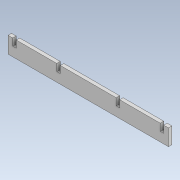
# Autodesk Inventor part: chassis_1_7
Saved by Autodesk Inventor 2022 (Build 260153000, 153)
## iProperties
Created: 2023-04-28
Part Number: chassis_1_7
Material: 一般
Document SubType Name: Modeling
Designer: Johnny Jou
Density: 1 g/cm^3
Appearance: 預設
Author: Johnny Jou
Autodesk Inventor part; units mm, degrees
ref_plane "YZ Plane" through (0, 0, 0) normal (1, 0, 0) x (0, 1, 0)
ref_plane "XZ Plane" through (0, 0, 0) normal (0, 1, 0) x (-1, 0, 0)
ref_plane "XY Plane" through (0, 0, 0) normal (0, 0, 1) x (1, 0, 0)
sketch "草圖1" plane through (0, 0, 0) normal (0, 0, 1) x (1, 0, 0)
  line L0 (0, 0) -> (124, 0)
  line L1 (124, 0) -> (124, -14) construction
  line L2 (124, -14) -> (0, -14)
  line L3 (0, -14) -> (0, 0) construction
  line L4 (35, 0) -> (37.95, 0)
  line L5 (37.95, 0) -> (37.95, -6)
  line L6 (37.95, -6) -> (35, -6)
  line L7 (35, -6) -> (35, 0)
  line L8 (89, 0) -> (86.05, 0)
  line L9 (86.05, 0) -> (86.05, -6)
  line L10 (86.05, -6) -> (89, -6)
  line L11 (89, -6) -> (89, 0)
  line L12 (131, -14) -> (126.95, -14)
  line L13 (124, 0) -> (131, 0)
  line L14 (131, 0) -> (131, -14)
  line L15 (126.95, -14) -> (126.95, -6)
  line L16 (126.95, -6) -> (124, -6)
  line L17 (0, 0) -> (-7, 0)
  line L18 (-7, 0) -> (-7, -14)
  line L19 (-7, -14) -> (-2.95, -14)
  line L20 (0, -14) -> (0, 0) construction
  line L21 (-2.95, -14) -> (-2.95, -6)
  line L22 (-2.95, -6) -> (0, -6)
  line L23 (0, -6) -> (0, -14)
  line L24 (124, -6) -> (124, -14)
  line L25 (124, -14) -> (126.95, -14)
  line L26 (124, -6) -> (126.95, -6)
  line L27 (126.95, -6) -> (126.95, 0)
  line L28 (126.95, 0) -> (124, 0)
  line L29 (124, 0) -> (124, -6)
  line L30 (-2.95, -14) -> (0, -14)
  line L31 (-2.95, -6) -> (0, -6)
  line L32 (0, -6) -> (0, 0)
  line L33 (0, 0) -> (-2.95, 0)
  line L34 (-2.95, 0) -> (-2.95, -6)
  point P0 (0, -15.5)
  point P1 (0, -6)
  point P2 (0, -14)
  dimension "d0" = 124
  dimension "d1" = 35
  dimension "d3" = 2.95
  dimension "d4" = 2.95
  dimension "d10" = 8
  dimension "d16" = 6
  dimension "d17" = 35
  dimension "d18" = 2.95
  dimension "d21" = 7
  dimension "d22" = 2.95
  dimension "d24" = 7
  dimension "d29" = 6
  dimension "d30" = 6
  constraints: 70 end point, 14 parallel, 8 horizontal, 8 perpendicular, 6 point on line, 4 collinear
  measures "d0" distance of L1.end L2.end
  measures "d1" distance between parallel lines of L3 L7
  measures "d3" distance of L5.end L6.end
  measures "d4" distance of L9.end L10.end
  measures "d10" distance between parallel lines of L2 L6
  measures "d16" distance of L6.end L4.start
  measures "d17" distance between parallel lines of L1 L11
  measures "d18" distance between parallel lines of L3 L21
  measures "d21" distance between parallel lines of L18 L3
  measures "d22" distance between parallel lines of L1 L15
  measures "d24" distance between parallel lines of L1 L14
  measures "d29" distance between parallel lines of L13 L16
  measures "d30" distance between parallel lines of L33 L31
extrude "擠出1" add sketch "草圖1" along normal blind 3 contours L0 L7 L6 L5 L9 L10 L11 L29 L24 L2 L23 L32 | L34 L21 L19 L18 L17 | L23 L30 L21 L22 | L24 L16 L15 L25 | L15 L27 L13 L14 L12
